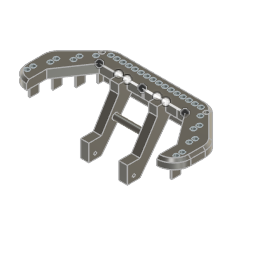
IR Sensor front (Autodesk Fusion 360 design; units mm, degrees)
part number: 2026-02-09-01-24-13-625
Autodesk Fusion 360 part; units mm, degrees
note: some values were not read from the file. Set by a fixed rule: which sketch regions a step uses.
sketch "Sketch1" plane through (0, 0, 0) normal (0, 0, 1) x (1, 0, 0)
  line L0 (0.0284, 49.9803) -> (112.0284, 49.9803)
  line L1 (0.0284, 49.9803) -> (14, 49.9848)
  line L2 (34, 49.9803) -> (35, 49.9803)
  line L3 (0.0284, 49.9803) -> (3.5, 49.981)
  circle A0 centre (3.5, 40) radius 2.5
  circle A1 centre (10.5, 40) radius 2.5
  circle A2 centre (17.5, 40) radius 2.5
  circle A3 centre (24.5, 40) radius 2.5
  circle A4 centre (52.5, 40) radius 2.5
  circle A5 centre (45.5, 40) radius 2.5
  circle A6 centre (38.5, 40) radius 2.5
  circle A7 centre (31.5, 40) radius 2.5
  circle A8 centre (80.5, 40) radius 2.5
  circle A9 centre (66.5, 40) radius 2.5
  circle A10 centre (87.5, 40) radius 2.5
  circle A11 centre (108.5, 40) radius 2.5
  circle A12 centre (101.5, 40) radius 2.5
  circle A13 centre (59.5, 40) radius 2.5
  circle A14 centre (73.5, 40) radius 2.5
  circle A15 centre (94.5, 40) radius 2.5
  line L4 (0.0284, 49.9803) -> (112, 49.9803)
  line L5 (0.0284, 35) -> (18.4391, 35) construction
  line L6 (0.0284, 49.9803) -> (21.4009, 49.9803) construction
  line L7 (0.0284, 49.9803) -> (17.8045, 49.9803) construction
  line L8 (0.0284, 35) -> (16.4184, 35) construction
  line L9 (0.0284, 35) -> (26.651, 35) construction
  line L10 (0.0284, 35) -> (21.4009, 35) construction
  line L11 (0.0284, 49.9803) -> (16.9706, 49.9803) construction
  line L12 (0.0284, 49.9803) -> (-39.8611, 10.0907)
  line L13 (-39.8611, 10.0907) -> (-39.8327, 0)
  line L14 (-39.8327, 0) -> (-39.734, -35)
  line L15 (16.4256, 25) -> (55, 25)
  line L16 (55, 25) -> (56, 25)
  line L17 (-19.9417, -11.3673) -> (-19.9417, -35)
  line L18 (-39.9417, -35) -> (-19.9417, -35)
  line L19 (-19.9417, -11.3673) -> (16.4256, 25)
  line L20 (-19.9417, -11.3673) -> (31.4894, -11.3673) construction
  line L21 (131.9417, -11.3673) -> (95.5744, 25)
  line L22 (111.9716, 49.9803) -> (98, 49.9848)
  line L23 (111.9716, 49.9803) -> (108.5, 49.981)
  line L24 (151.9417, -35) -> (131.9417, -35)
  line L25 (151.8611, 10.0907) -> (151.8327, 0)
  line L26 (78, 49.9803) -> (77, 49.9803)
  line L27 (151.8327, 0) -> (151.8327, -15)
  line L28 (57, 25) -> (56, 25)
  circle A16 centre (59.5, 40) radius 2.5
  circle A17 centre (87.5, 40) radius 2.5
  line L29 (111.9716, 49.9803) -> (95.0294, 49.9803) construction
  circle A18 centre (66.5, 40) radius 2.5
  circle A19 centre (80.5, 40) radius 2.5
  circle A20 centre (108.5, 40) radius 2.5
  line L30 (111.9716, 49.9803) -> (151.8611, 10.0907)
  line L31 (131.9417, -11.3673) -> (131.9417, -35)
  line L32 (111.9716, 49.9803) -> (94.1955, 49.9803) construction
  circle A21 centre (101.5, 40) radius 2.5
  line L33 (111.9716, 35) -> (95.5816, 35) construction
  line L34 (95.5744, 25) -> (57, 25)
  line L35 (131.9417, -11.3673) -> (80.5106, -11.3673) construction
  circle A22 centre (94.5, 40) radius 2.5
  line L36 (111.9716, 35) -> (90.5991, 35) construction
  circle A23 centre (73.5, 40) radius 2.5
  line L37 (111.9716, 49.9803) -> (90.5991, 49.9803) construction
  line L38 (151.8611, 10.0908) -> (151.8327, 0)
  line L39 (151.8327, 0) -> (151.734, -35)
  line L40 (-10.0048, 29.3243) -> (4.6262, 29.3243) construction
  line L41 (-4.8319, 34.4971) -> (-4.8319, 35.4971)
  line L42 (-4.8319, 35.4971) -> (-4.8319, 37.9971)
  circle A24 centre (-4.8319, 37.9971) radius 2.5
  circle A25 centre (-4.8319, 30.9971) radius 2.5
  line L43 (-19.9163, 19.3711) -> (-5.8699, 19.3711) construction
  line L44 (-9.984, 29.3034) -> (4.3283, 29.3034) construction
  circle A26 centre (-24.9502, -2.1627) radius 2.5
  circle A27 centre (-24.9502, 4.8373) radius 2.5
  circle A28 centre (-30.9502, -16.1627) radius 2.5
  circle A29 centre (-30.9502, -23.1627) radius 2.5
  circle A30 centre (-13.9502, 20.8373) radius 2.5
  circle A31 centre (-13.9502, 13.8373) radius 2.5
  circle A32 centre (116.8319, 37.9971) radius 2.5
  circle A33 centre (116.8319, 30.9971) radius 2.5
  line L45 (116.8319, 35.4971) -> (116.8319, 37.9971)
  line L46 (151.8327, 0) -> (151.734, -35)
  line L47 (116.8319, 34.4971) -> (116.8319, 35.4971)
  line L48 (131.9417, -11.3673) -> (131.9417, -35)
  circle A34 centre (142.9502, -23.1627) radius 2.5
  line L49 (151.9417, -35) -> (131.9417, -35)
  circle A35 centre (136.9502, 4.8373) radius 2.5
  circle A36 centre (125.9502, 20.8373) radius 2.5
  circle A37 centre (142.9502, -16.1627) radius 2.5
  line L50 (131.9163, 19.3711) -> (117.8699, 19.3711) construction
  line L51 (151.8611, 10.0907) -> (151.8327, 0)
  circle A38 centre (125.9502, 13.8373) radius 2.5
  circle A39 centre (136.9502, -2.1627) radius 2.5
  point P0 (151.9417, -35)
  point P1 (121.984, 29.3034)
  point P2 (122.0048, 29.3243)
  dimension "d1" = 112
  dimension "d40" = 45
  dimension "d42" = 1
  dimension "d43" = 2.5
  dimension "d44" = 5
  constraint horizontal L0
  constraint coincident L0 L2.start
  constraint coincident L0 L2.end
  constraint horizontal L4
  constraint horizontal L5
  constraint horizontal L6
  constraint horizontal L7
  constraint horizontal L8
  constraint horizontal L9
  constraint horizontal L10
  constraint horizontal L11
  constraint parallel L13 L14
  constraint perpendicular L17 L18
  constraint horizontal L20
  constraint coincident L18 L14.end
  constraint horizontal L40
  constraint vertical L41
  constraint parallel L41 L42
  constraint coincident L42.end A24.centre
  constraint horizontal L43
  constraint horizontal L44
  measures "d1" distance of L0.start L0.end
  measures "d40" angle of L19 L20
  measures "d42" distance of L41.start L41.end
  measures "d43" distance of L41.end L42.end
  measures "d44" diameter of A24
sketch "Sketch2" plane through (0, 0, 0) normal (0, 0, 1) x (1, 0, 0)
extrude "Extrude1" add sketch "Sketch1" against normal blind 10
fillet "Fillet1" radius 20 6 edges at (151.8611, 10.0907, -5) (151.734, -35, -5) (111.9716, 49.9803, -5) (0.0284, 49.9803, -5) (-39.8611, 10.0907, -5) (-39.734, -35, -5)
sketch "Sketch3" plane through (0, 0, 0) normal (0, 0, 1) x (1, 0, 0)
chamfer "Chamfer1" distance 3 angle 45 13 edges at (42.6564, 49.9803, 0) (77.5, 49.9803, 0) (90.8436, 49.9803, 0) (111.341, 48.4579, 0) (131.9047, 30.0472, 0) (150.3261, 9.4575, 0) (151.814, -6.6417, 0) (145.966, -29.1091, 0) (-33.966, -29.1091, 0) (-39.814, -6.6417, 0) (-38.3261, 9.4575, 0) (-19.9047, 30.0472, 0) (0.659, 48.4579, 0)
sketch "Sketch4" plane through (0, 0, 0) normal (0, 0, 1) x (1, 0, 0)
  line L0 (131.9417, -11.3672) -> (105, 25)
  line L1 (105, 25) -> (5, 25)
  line L2 (5, 25) -> (-19.9417, -11.3672)
  line L3 (-19.9417, -11.3672) -> (131.9417, -11.3672)
  constraint horizontal L1
extrude "Extrude2" cut sketch "Sketch4" against normal blind 10
move_face "OffsetFaces1" offset -0.3 32 faces at (-28.4533, -23.2873, -6.6667) (-28.4533, -16.2873, -6.6667) (-22.4533, -2.2873, -6.6667) (-22.4533, 4.7127, -6.6667) (-11.4533, 13.7127, -6.6667) (-11.4533, 20.7127, -6.6667) (-2.3351, 30.8725, -6.6667) (-5.5688, 35.6082, -6.6667) (5.9969, 39.8754, -6.6667) (12.9969, 39.8754, -6.6667) (19.9969, 39.8754, -6.6667) (26.9969, 39.8754, -6.6667) (33.9969, 39.8754, -6.6667) (40.9969, 39.8754, -6.6667) (47.9969, 39.8754, -6.6667) (54.9969, 39.8754, -6.6667) (61.9969, 39.8754, -6.6667) (68.9969, 39.8754, -6.6667) (75.9969, 39.8754, -6.6667) (82.9969, 39.8754, -6.6667) (89.9969, 39.8754, -6.6667) (96.9969, 39.8754, -6.6667) (103.9969, 39.8754, -6.6667) (110.9969, 39.8754, -6.6667) (117.2186, 40.467, -6.6667) (119.3288, 30.8725, -6.6667) (128.4471, 13.7127, -6.6667) (128.4471, 20.7127, -6.6667) (137.6273, 7.2438, -6.6667) (137.6273, 0.2438, -6.6667) (143.6273, -13.7562, -6.6667) (143.6273, -20.7562, -6.6667)
sketch "Sketch5" plane through (0, 0, 0) normal (0, 0, 1) x (1, 0, 0)
sketch "Sketch6" plane through (0, 0, 0) normal (1, 0, 0) x (0, 1, 0)
sketch "Sketch7" plane through (0, 0, 0) normal (0, 0, 1) x (1, 0, 0)
sketch "Sketch8" plane through (0, 0, 0) normal (1, 0, 0) x (0, 1, 0)
sketch "Sketch9" plane through (0, 0, -10) normal (0, 0, -1) x (1, 0, 0)
  circle A0 centre (3.5, -40) radius 2.8
  circle A1 centre (136.9502, -4.8373) radius 2.8
  circle A2 centre (-13.9502, -13.8373) radius 2.8
  circle A3 centre (17.5, -40) radius 2.8
  circle A4 centre (142.9502, 23.1627) radius 2.8
  circle A5 centre (-24.9502, -4.8373) radius 2.8
  circle A6 centre (-13.9502, -20.8373) radius 2.8
  circle A7 centre (73.5, -40) radius 2.8
  circle A8 centre (52.5, -40) radius 2.8
  circle A9 centre (116.8319, -37.9971) radius 2.8
  circle A10 centre (-4.8319, -37.9971) radius 2.8
  circle A11 centre (45.5, -40) radius 2.8
  circle A12 centre (136.9502, 2.1627) radius 2.8
  circle A13 centre (10.5, -40) radius 2.8
  circle A14 centre (-30.9502, 23.1627) radius 2.8
  circle A15 centre (116.8319, -30.9971) radius 2.8
  circle A16 centre (66.5, -40) radius 2.8
  circle A17 centre (24.5, -40) radius 2.8
  circle A18 centre (108.5, -40) radius 2.8
  circle A19 centre (-4.8319, -30.9971) radius 2.8
  circle A20 centre (142.9502, 16.1627) radius 2.8
  circle A21 centre (94.5, -40) radius 2.8
  circle A22 centre (125.9502, -20.8373) radius 2.8
  circle A23 centre (59.5, -40) radius 2.8
  circle A24 centre (31.5, -40) radius 2.8
  circle A25 centre (101.5, -40) radius 2.8
  circle A26 centre (125.9502, -13.8373) radius 2.8
  circle A27 centre (-24.9502, 2.1627) radius 2.8
  circle A28 centre (80.5, -40) radius 2.8
  circle A29 centre (87.5, -40) radius 2.8
  circle A30 centre (38.5, -40) radius 2.8
  circle A31 centre (-30.9502, 16.1627) radius 2.8
  line L0 (131.9417, 11.3673) -> (105, -25)
  line L1 (105, -25) -> (95.5744, -25)
  line L2 (95.5744, -25) -> (57, -25)
  line L3 (57, -25) -> (55, -25)
  line L4 (55, -25) -> (5, -25)
  line L5 (5, -25) -> (-19.9417, 11.3672)
  line L6 (-19.9417, 11.3673) -> (-19.9417, 35)
  arc A32 (-19.9417, 35) -> (-39.7902, 15.057) centre (-19.7903, 15.0006) ccw
  line L7 (-39.7902, 15.057) -> (-39.8377, -1.7735)
  arc A33 (-39.8377, -1.7735) -> (-33.9799, -15.972) centre (-19.8378, -1.8298) ccw
  line L8 (-33.9799, -15.972) -> (-5.8294, -44.1225)
  arc A34 (-5.8294, -44.1225) -> (8.3127, -49.9803) centre (8.3127, -29.9803) ccw
  line L9 (8.3127, -49.9803) -> (77, -49.9803)
  line L10 (77, -49.9803) -> (78, -49.9803)
  line L11 (78, -49.9803) -> (103.6873, -49.9803)
  arc A35 (103.6873, -49.9803) -> (117.8294, -44.1225) centre (103.6873, -29.9803) ccw
  line L12 (117.8294, -44.1225) -> (145.9799, -15.972)
  arc A36 (145.9799, -15.972) -> (151.8377, -1.7735) centre (131.8378, -1.8298) ccw
  line L13 (151.8377, -1.7735) -> (151.7902, 15.057)
  arc A37 (151.7902, 15.057) -> (131.9417, 35) centre (131.7903, 15.0006) ccw
  line L14 (131.9417, 35) -> (131.9417, 11.3673)
  line L15 (111.7359, -34.6155) -> (0, -34.6155)
  line L16 (111.7359, -36.6155) -> (0, -36.6155)
  line L17 (113.7359, -39.4874) -> (113.7359, -28.7703)
  line L18 (111.7359, -39.483) -> (111.7359, -28.6527)
  line L19 (122.7359, -22.5163) -> (122.7359, -11.7992)
  line L20 (120.7359, -22.5119) -> (120.7359, -11.6815)
  line L21 (131.7359, -6.4947) -> (131.7359, 4.3357)
  line L22 (133.7359, -6.4991) -> (133.7359, 4.218)
  line L23 (137.7359, 14.5053) -> (137.7359, 25.3357)
  line L24 (139.7359, 14.5009) -> (139.7359, 25.218)
  line L25 (139.7359, 14.5009) -> (137.7359, 14.5053)
  line L26 (137.7359, 25.3357) -> (139.7359, 25.218)
  line L27 (133.7359, 4.218) -> (131.7359, 4.3357)
  line L28 (131.7359, -6.4947) -> (133.7359, -6.4991)
  line L29 (122.7359, -11.7992) -> (120.7359, -11.6815)
  line L30 (120.7359, -22.5119) -> (122.7359, -22.5163)
  line L31 (113.7359, -28.7703) -> (111.7359, -28.6527)
  line L32 (113.7359, -39.4874) -> (111.7359, -39.483)
  line L33 (56.7001, -39.9767) -> (55.2999, -39.9767)
  line L34 (56, -39.9767) -> (56, -24)
  line L35 (-25.7359, 14.5053) -> (-25.7359, 25.3357)
  line L36 (-27.7359, 14.5009) -> (-27.7359, 25.218)
  line L37 (-27.7359, 14.5009) -> (-25.7359, 14.5053)
  line L38 (-25.7359, 25.3357) -> (-27.7359, 25.218)
  line L39 (-19.7359, -6.4947) -> (-21.7359, -6.4991)
  line L40 (-19.7359, -6.4947) -> (-19.7359, 4.3357)
  line L41 (-21.7359, -6.4991) -> (-21.7359, 4.218)
  line L42 (-21.7359, 4.218) -> (-19.7359, 4.3357)
  line L43 (-8.7359, -22.5119) -> (-8.7359, -11.6815)
  line L44 (-10.7359, -11.7992) -> (-8.7359, -11.6815)
  line L45 (-10.7359, -22.5163) -> (-10.7359, -11.7992)
  line L46 (-8.7359, -22.5119) -> (-10.7359, -22.5163)
  line L47 (0.2641, -39.9767) -> (0.2641, -28.6527)
  line L48 (-1.7359, -28.7703) -> (0.2641, -28.6527)
  line L49 (-1.7359, -39.4874) -> (-1.7359, -28.7703)
  line L50 (-1.7359, -39.4874) -> (0.2641, -39.483)
  dimension "d63" = 2
  dimension "d64" = 2
  dimension "d65" = 2
  constraint horizontal L15
  constraint vertical L17
  constraint coincident L18 L15.start
  constraint vertical L19
  constraint vertical L22
  constraint vertical L24
  constraint parallel L26 L27
  constraint coincident A23 L33.start
  constraint coincident A8 L33.end
  constraint horizontal L33
  constraint midpoint L33 L34.start
  constraint perpendicular L3 L34
  constraint symmetric L17.end L34 L48.start
  constraint symmetric L18.start L34 L50.end
  constraint symmetric L18.end L34 L47.end
  constraint symmetric L17.start L34 L49.start
  constraint symmetric L19.end L34 L44.start
  constraint symmetric L19.start L34 L45.start
  constraint symmetric L20.start L34 L43.start
  constraint symmetric L20.end L34 L43.end
  constraint symmetric L21.start L34 L39.start
  constraint symmetric L21.end L34 L40.end
  constraint symmetric L22.end L34 L41.end
  constraint symmetric L22.start L34 L39.end
  constraint symmetric L24.start L34 L36.start
  constraint symmetric L23.start L34 L35.start
  constraint symmetric L23.end L34 L35.end
  constraint symmetric L24.end L34 L36.end
  constraint coincident L50.end L47
  constraint coincident L18 L16.start
  measures "d63" distance of L19 L20
  measures "d64" distance of L21 L22
  measures "d65" distance of L23 L24
extrude "Extrude3" add sketch "Sketch9" along normal blind 15 contours L15 L16 L18 L34 | L17 L18 L31 L32 | L15 L16 L34 L47 | L47 L48 L49 L50 | L19 L20 L29 L30 | L21 L22 L27 L28 | L23 L24 L25 L26 | L35 L36 L37 L38 | L39 L40 L41 L42 | L43 L44 L45 L46
sketch "Sketch10" plane through (0, 0, 0) normal (0, 0, 1) x (-1, 0, 0)
  line L0 (-105, -25) -> (-131.9417, 11.3673)
  line L1 (-131.9417, 11.3673) -> (-131.9417, 31.9999)
  arc A0 (-131.9417, 31.9999) -> (-148.7902, 15.0485) centre (-131.7903, 15.0006) ccw
  line L2 (-148.7902, 15.0485) -> (-148.8377, -1.7819)
  arc A1 (-148.8377, -1.7819) -> (-143.8586, -13.8507) centre (-131.8378, -1.8298) ccw
  line L3 (-143.8586, -13.8507) -> (-119.6308, -38.0785)
  arc A2 (-116.9133, -40.7959) -> (-119.6308, -38.0785) centre (-116.8319, -37.9971) ccw
  line L4 (-116.9133, -40.7959) -> (-115.7081, -42.0011)
  arc A3 (-115.7081, -42.0011) -> (-103.6873, -46.9803) centre (-103.6873, -29.9803) ccw
  line L5 (-103.6873, -46.9803) -> (-78, -46.9803)
  line L6 (-78, -46.9803) -> (-77, -46.9803)
  line L7 (-77, -46.9803) -> (-8.3127, -46.9803)
  arc A4 (-8.3127, -46.9803) -> (3.7081, -42.0011) centre (-8.3127, -29.9803) ccw
  line L8 (3.7081, -42.0011) -> (4.9133, -40.7959)
  arc A5 (7.6308, -38.0785) -> (4.9133, -40.7959) centre (4.8319, -37.9971) ccw
  line L9 (7.6308, -38.0785) -> (31.8586, -13.8507)
  arc A6 (31.8586, -13.8507) -> (36.8377, -1.7819) centre (19.8378, -1.8298) ccw
  line L10 (36.8377, -1.7819) -> (36.7902, 15.0485)
  arc A7 (36.7902, 15.0485) -> (19.9417, 31.9999) centre (19.7903, 15.0006) ccw
  line L11 (19.9417, 31.9999) -> (19.9417, 11.3673)
  line L12 (19.9417, 11.3672) -> (-5, -25)
  line L13 (-5, -25) -> (-55, -25)
  line L14 (-55, -25) -> (-57, -25)
  line L15 (-57, -25) -> (-95.5744, -25)
  line L16 (-95.5744, -25) -> (-105, -25)
  circle A8 centre (30.9502, 16.1627) radius 2.8
  circle A9 centre (-38.5, -40) radius 2.8
  circle A10 centre (-87.5, -40) radius 2.8
  circle A11 centre (-80.5, -40) radius 2.8
  circle A12 centre (24.9502, 2.1627) radius 2.8
  circle A13 centre (-125.9502, -13.8373) radius 2.8
  circle A14 centre (-101.5, -40) radius 2.8
  circle A15 centre (-31.5, -40) radius 2.8
  circle A16 centre (-59.5, -40) radius 2.8
  circle A17 centre (-125.9502, -20.8373) radius 2.8
  circle A18 centre (-94.5, -40) radius 2.8
  circle A19 centre (-142.9502, 16.1627) radius 2.8
  circle A20 centre (4.8319, -30.9971) radius 2.8
  circle A21 centre (-108.5, -40) radius 2.8
  circle A22 centre (-24.5, -40) radius 2.8
  circle A23 centre (-66.5, -40) radius 2.8
  circle A24 centre (-116.8319, -30.9971) radius 2.8
  circle A25 centre (30.9502, 23.1627) radius 2.8
  circle A26 centre (-10.5, -40) radius 2.8
  circle A27 centre (-136.9502, 2.1627) radius 2.8
  circle A28 centre (-45.5, -40) radius 2.8
  circle A29 centre (-52.5, -40) radius 2.8
  circle A30 centre (-73.5, -40) radius 2.8
  circle A31 centre (13.9502, -20.8373) radius 2.8
  circle A32 centre (24.9502, -4.8373) radius 2.8
  circle A33 centre (-142.9502, 23.1627) radius 2.8
  circle A34 centre (-17.5, -40) radius 2.8
  circle A35 centre (13.9502, -13.8373) radius 2.8
  circle A36 centre (-136.9502, -4.8373) radius 2.8
  circle A37 centre (-3.5, -40) radius 2.8
  line L17 (-5, -25) -> (-105, -25)
  line L18 (-105, -25) -> (-55, -25)
  line L19 (-55, -25) -> (-27.5, -25)
  line L20 (-55, -25) -> (-37.5, -25)
  line L21 (-55, -25) -> (-72.5, -25)
  line L22 (-55, -25) -> (-82.5, -25)
  dimension "d68" = 50
  dimension "d69" = 27.5
  dimension "d70" = 17.5
  dimension "d71" = 17.5
  dimension "d72" = 27.5
  constraint coincident L12.end L13.start
  constraint coincident L0.start L16.end
  constraint parallel L17 L18
  constraint parallel L17 L19
  constraint coincident L13.end L14.start
  constraint parallel L19 L20
  constraint parallel L15 L21
  constraint parallel L17 L22
  measures "d68" distance of L0.start L13.end
  measures "d69" distance of L13.end L19.end
  measures "d70" distance of L13.end L20.end
  measures "d71" distance of L13.end L21.end
  measures "d72" distance of L13.end L22.end
sketch "Sketch11" plane through (0, 25, 0) normal (0, -1, 0) x (1, 0, 0)
  line L0 (95.5744, 0) -> (57, 0)
  line L1 (57, 0) -> (57, -10)
  line L2 (57, -10) -> (95.5744, -10)
  line L3 (95.5744, -10) -> (95.5744, 0)
  line L4 (82.5, 0) -> (72.5, 0)
  line L5 (72.5, 0) -> (72.5, -10)
  line L6 (72.5, -10) -> (82.5, -10)
  line L7 (82.5, -10) -> (82.5, 0)
  line L8 (37.5, 0) -> (27.5, 0)
  line L9 (27.5, 0) -> (27.5, -10)
  line L10 (27.5, -10) -> (37.5, -10)
  line L11 (37.5, -10) -> (37.5, 0)
  point P0 (82.5, 0)
  point P1 (72.5, 0)
  point P2 (37.5, 0)
  point P3 (27.5, 0)
  dimension "d73" = 10
  dimension "d74" = 10
  dimension "d75" = 10
  dimension "d76" = 10
  constraint horizontal L4
  constraint vertical L5
  constraint horizontal L6
  constraint vertical L7
  constraint coincident P0 L4.start
  constraint horizontal L8
  constraint vertical L9
  constraint horizontal L10
  constraint vertical L11
  constraint coincident P2 L8.start
  measures "d73" distance of P0 P1
  measures "d74" distance of P0 L6.end
  measures "d75" distance of P2 P3
  measures "d76" distance of P2 L10.end
ref_plane "WorkPlane1" through (30, -5, -5) normal (0, -1, 0) x (-1, 0, 0)
sketch "Sketch12" plane through (0, -5, 0) normal (0, -1, 0) x (-1, 0, 0)
  line L0 (-37.5, 42) -> (-27.9, 42)
  line L1 (-27.9, 42) -> (-27.9, 62)
  line L2 (-27.9, 62) -> (-37.5, 62)
  line L3 (-37.5, 62) -> (-37.5, 42)
  point P0 (-72.5, 0)
  point P1 (-82.5, 0)
  point P2 (-27.5, 0)
  point P3 (-37.5, 0)
  dimension "d81" = 42
  dimension "d82" = 9.6
  dimension "d83" = 20
  constraint horizontal L0
  constraint vertical L1
  constraint horizontal L2
  constraint vertical L3
  measures "d81" distance of P3 L0.start
  measures "d82" distance of L0.start L0.end
  measures "d83" distance of L0.start L2.end
extrude "Extrude4" add sketch "Sketch11" along normal blind 10 contours L0 L2 L4 L5 L6 L7 | L8 L9 L10 L11
sketch "Sketch13" plane through (0, 0, -10) normal (0, 0, -1) x (1, 0, 0)
  line L0 (-27.7359, 14.5009) -> (-27.7359, 25.218)
  line L1 (-27.7359, 25.218) -> (-25.7359, 25.3357)
  line L2 (-25.7359, 25.3357) -> (-25.7359, 14.5053)
  line L3 (-25.7359, 14.5053) -> (-27.7359, 14.5009)
  line L4 (131.7359, -6.4947) -> (131.7359, 4.3357)
  line L5 (131.7359, 4.3357) -> (133.7359, 4.218)
  line L6 (133.7359, 4.218) -> (133.7359, -6.4991)
  line L7 (133.7359, -6.4991) -> (131.7359, -6.4947)
  line L8 (120.7359, -22.5119) -> (120.7359, -11.6815)
  line L9 (120.7359, -11.6815) -> (122.7359, -11.7992)
  line L10 (122.7359, -11.7992) -> (122.7359, -22.5163)
  line L11 (122.7359, -22.5163) -> (120.7359, -22.5119)
  line L12 (-19.7359, -6.4947) -> (-21.7359, -6.4991)
  line L13 (-21.7359, -6.4991) -> (-21.7359, 4.218)
  line L14 (-21.7359, 4.218) -> (-19.7359, 4.3357)
  line L15 (-19.7359, 4.3357) -> (-19.7359, -6.4947)
  line L16 (139.7359, 14.5009) -> (137.7359, 14.5053)
  line L17 (137.7359, 14.5053) -> (137.7359, 25.3357)
  line L18 (137.7359, 25.3357) -> (139.7359, 25.218)
  line L19 (139.7359, 25.218) -> (139.7359, 14.5009)
  line L20 (-1.7359, -28.7703) -> (0.2641, -28.6527)
  line L21 (0.2641, -28.6527) -> (0.2641, -34.6155)
  line L22 (0.2641, -34.6155) -> (111.7359, -34.6155)
  line L23 (111.7359, -34.6155) -> (111.7359, -28.6527)
  line L24 (111.7359, -28.6527) -> (113.7359, -28.7703)
  line L25 (113.7359, -28.7703) -> (113.7359, -39.4874)
  line L26 (113.7359, -39.4874) -> (111.7359, -39.483)
  line L27 (111.7359, -39.483) -> (111.7359, -36.6155)
  line L28 (111.7359, -36.6155) -> (0.2641, -36.6155)
  line L29 (0.2641, -36.6155) -> (0.2641, -39.483)
  line L30 (0.2641, -39.483) -> (-1.7359, -39.4874)
  line L31 (-1.7359, -39.4874) -> (-1.7359, -28.7703)
  line L32 (-8.7359, -22.5119) -> (-10.7359, -22.5163)
  line L33 (-10.7359, -22.5163) -> (-10.7359, -11.7992)
  line L34 (-10.7359, -11.7992) -> (-8.7359, -11.6815)
  line L35 (-8.7359, -11.6815) -> (-8.7359, -22.5119)
  circle A0 centre (3.5, -40) radius 2.8
  circle A1 centre (136.9502, -4.8373) radius 2.8
  circle A2 centre (-13.9502, -13.8373) radius 2.8
  circle A3 centre (17.5, -40) radius 2.8
  circle A4 centre (142.9502, 23.1627) radius 2.8
  circle A5 centre (-24.9502, -4.8373) radius 2.8
  circle A6 centre (-13.9502, -20.8373) radius 2.8
  circle A7 centre (73.5, -40) radius 2.8
  circle A8 centre (52.5, -40) radius 2.8
  circle A9 centre (116.8319, -37.9971) radius 2.8
  circle A10 centre (-4.8319, -37.9971) radius 2.8
  circle A11 centre (45.5, -40) radius 2.8
  circle A12 centre (136.9502, 2.1627) radius 2.8
  circle A13 centre (10.5, -40) radius 2.8
  circle A14 centre (-30.9502, 23.1627) radius 2.8
  circle A15 centre (116.8319, -30.9971) radius 2.8
  circle A16 centre (66.5, -40) radius 2.8
  circle A17 centre (24.5, -40) radius 2.8
  circle A18 centre (108.5, -40) radius 2.8
  circle A19 centre (-4.8319, -30.9971) radius 2.8
  circle A20 centre (142.9502, 16.1627) radius 2.8
  circle A21 centre (94.5, -40) radius 2.8
  circle A22 centre (125.9502, -20.8373) radius 2.8
  circle A23 centre (59.5, -40) radius 2.8
  circle A24 centre (31.5, -40) radius 2.8
  circle A25 centre (101.5, -40) radius 2.8
  circle A26 centre (125.9502, -13.8373) radius 2.8
  circle A27 centre (-24.9502, 2.1627) radius 2.8
  circle A28 centre (80.5, -40) radius 2.8
  circle A29 centre (87.5, -40) radius 2.8
  circle A30 centre (38.5, -40) radius 2.8
  circle A31 centre (-30.9502, 16.1627) radius 2.8
  line L36 (131.9417, 11.3673) -> (105, -25)
  line L37 (105, -25) -> (95.5744, -25)
  line L38 (95.5744, -25) -> (82.5, -25)
  line L39 (82.5, -25) -> (82.5, -15)
  line L40 (82.5, -15) -> (72.5, -15)
  line L41 (72.5, -15) -> (72.5, -25)
  line L42 (72.5, -25) -> (57, -25)
  line L43 (57, -25) -> (55, -25)
  line L44 (55, -25) -> (37.5, -25)
  line L45 (37.5, -25) -> (37.5, -15)
  line L46 (37.5, -15) -> (27.5, -15)
  line L47 (27.5, -15) -> (27.5, -25)
  line L48 (27.5, -25) -> (5, -25)
  line L49 (5, -25) -> (-19.9417, 11.3672)
  line L50 (-19.9417, 11.3673) -> (-19.9417, 35)
  arc A32 (-19.9417, 35) -> (-39.7902, 15.057) centre (-19.7903, 15.0006) ccw
  line L51 (-39.7902, 15.057) -> (-39.8377, -1.7735)
  arc A33 (-39.8377, -1.7735) -> (-33.9799, -15.972) centre (-19.8378, -1.8298) ccw
  line L52 (-33.9799, -15.972) -> (-5.8294, -44.1225)
  arc A34 (-5.8294, -44.1225) -> (8.3127, -49.9803) centre (8.3127, -29.9803) ccw
  line L53 (8.3127, -49.9803) -> (77, -49.9803)
  line L54 (77, -49.9803) -> (78, -49.9803)
  line L55 (78, -49.9803) -> (103.6873, -49.9803)
  arc A35 (103.6873, -49.9803) -> (117.8294, -44.1225) centre (103.6873, -29.9803) ccw
  line L56 (117.8294, -44.1225) -> (145.9799, -15.972)
  arc A36 (145.9799, -15.972) -> (151.8377, -1.7735) centre (131.8378, -1.8298) ccw
  line L57 (151.8377, -1.7735) -> (151.7902, 15.057)
  arc A37 (151.7902, 15.057) -> (131.9417, 35) centre (131.7903, 15.0006) ccw
  line L58 (131.9417, 35) -> (131.9417, 11.3673)
  line L59 (82.5, -15) -> (72.5, -15)
  line L60 (72.5, -15) -> (72.5, -34.6155)
  line L61 (72.5, -34.6155) -> (82.5, -34.6155)
  line L62 (82.5, -34.6155) -> (82.5, -15)
  line L63 (37.5, -15) -> (27.5, -15)
  line L64 (27.5, -15) -> (27.5, -34.6155)
  line L65 (27.5, -34.6155) -> (37.5, -34.6155)
  line L66 (37.5, -34.6155) -> (37.5, -15)
  dimension "d86" = 10
  dimension "d87" = 10
  constraint horizontal L59
  constraint vertical L60
  constraint horizontal L61
  constraint vertical L62
  constraint coincident L39.end L40.start
  constraint horizontal L63
  constraint vertical L64
  constraint horizontal L65
  constraint vertical L66
  constraint coincident L45.end L46.start
  measures "d86" distance of L39.end L40.end
  measures "d87" distance of L45.end L46.end
sketch "Sketch14" plane through (0, 0, -10) normal (0, 0, -1) x (1, 0, 0)
loft "Loft1" add profiles "Sketch13", "Sketch12" section 1 contours L22 L45 L46 L47 L63 L64 L65 L66 section 2
sketch "Sketch15" plane through (0, 0, -10) normal (0, 0, -1) x (1, 0, 0)
  circle A0 centre (-30.9502, 16.1627) radius 2.8
  circle A1 centre (38.5, -40) radius 2.8
  circle A2 centre (87.5, -40) radius 2.8
  circle A3 centre (80.5, -40) radius 2.8
  circle A4 centre (-24.9502, 2.1627) radius 2.8
  circle A5 centre (125.9502, -13.8373) radius 2.8
  circle A6 centre (101.5, -40) radius 2.8
  circle A7 centre (31.5, -40) radius 2.8
  circle A8 centre (59.5, -40) radius 2.8
  circle A9 centre (125.9502, -20.8373) radius 2.8
  circle A10 centre (94.5, -40) radius 2.8
  circle A11 centre (142.9502, 16.1627) radius 2.8
  circle A12 centre (-4.8319, -30.9971) radius 2.8
  circle A13 centre (108.5, -40) radius 2.8
  circle A14 centre (24.5, -40) radius 2.8
  circle A15 centre (66.5, -40) radius 2.8
  circle A16 centre (116.8319, -30.9971) radius 2.8
  circle A17 centre (-30.9502, 23.1627) radius 2.8
  circle A18 centre (10.5, -40) radius 2.8
  circle A19 centre (136.9502, 2.1627) radius 2.8
  circle A20 centre (45.5, -40) radius 2.8
  circle A21 centre (-4.8319, -37.9971) radius 2.8
  circle A22 centre (116.8319, -37.9971) radius 2.8
  circle A23 centre (52.5, -40) radius 2.8
  circle A24 centre (73.5, -40) radius 2.8
  circle A25 centre (-13.9502, -20.8373) radius 2.8
  circle A26 centre (-24.9502, -4.8373) radius 2.8
  circle A27 centre (142.9502, 23.1627) radius 2.8
  circle A28 centre (17.5, -40) radius 2.8
  circle A29 centre (-13.9502, -13.8373) radius 2.8
  circle A30 centre (136.9502, -4.8373) radius 2.8
  circle A31 centre (3.5, -40) radius 2.8
  line L0 (-8.7359, -22.5119) -> (-10.7359, -22.5163)
  line L1 (-10.7359, -22.5163) -> (-10.7359, -11.7992)
  line L2 (-10.7359, -11.7992) -> (-8.7359, -11.6815)
  line L3 (-8.7359, -11.6815) -> (-8.7359, -22.5119)
  line L4 (37.5, -25) -> (37.5, -34.6155)
  line L5 (37.5, -34.6155) -> (111.7359, -34.6155)
  line L6 (111.7359, -34.6155) -> (111.7359, -28.6527)
  line L7 (111.7359, -28.6527) -> (113.7359, -28.7703)
  line L8 (113.7359, -28.7703) -> (113.7359, -39.4874)
  line L9 (113.7359, -39.4874) -> (111.7359, -39.483)
  line L10 (111.7359, -39.483) -> (111.7359, -36.6155)
  line L11 (111.7359, -36.6155) -> (0.2641, -36.6155)
  line L12 (0.2641, -36.6155) -> (0.2641, -39.483)
  line L13 (0.2641, -39.483) -> (-1.7359, -39.4874)
  line L14 (-1.7359, -39.4874) -> (-1.7359, -28.7703)
  line L15 (-1.7359, -28.7703) -> (0.2641, -28.6527)
  line L16 (0.2641, -28.6527) -> (0.2641, -34.6155)
  line L17 (0.2641, -34.6155) -> (27.5, -34.6155)
  line L18 (27.5, -34.6155) -> (27.5, -25)
  line L19 (27.5, -25) -> (5, -25)
  line L20 (5, -25) -> (-19.9417, 11.3672)
  line L21 (-19.9417, 11.3673) -> (-19.9417, 35)
  arc A32 (-19.9417, 35) -> (-39.7902, 15.057) centre (-19.7903, 15.0006) ccw
  line L22 (-39.7902, 15.057) -> (-39.8377, -1.7735)
  arc A33 (-39.8377, -1.7735) -> (-33.9799, -15.972) centre (-19.8378, -1.8298) ccw
  line L23 (-33.9799, -15.972) -> (-5.8294, -44.1225)
  arc A34 (-5.8294, -44.1225) -> (8.3127, -49.9803) centre (8.3127, -29.9803) ccw
  line L24 (8.3127, -49.9803) -> (77, -49.9803)
  line L25 (77, -49.9803) -> (78, -49.9803)
  line L26 (78, -49.9803) -> (103.6873, -49.9803)
  arc A35 (103.6873, -49.9803) -> (117.8294, -44.1225) centre (103.6873, -29.9803) ccw
  line L27 (117.8294, -44.1225) -> (145.9799, -15.972)
  arc A36 (145.9799, -15.972) -> (151.8377, -1.7735) centre (131.8378, -1.8298) ccw
  line L28 (151.8377, -1.7735) -> (151.7902, 15.057)
  arc A37 (151.7902, 15.057) -> (131.9417, 35) centre (131.7903, 15.0006) ccw
  line L29 (131.9417, 35) -> (131.9417, 11.3673)
  line L30 (131.9417, 11.3673) -> (105, -25)
  line L31 (105, -25) -> (95.5744, -25)
  line L32 (95.5744, -25) -> (82.5, -25)
  line L33 (82.5, -25) -> (82.5, -15)
  line L34 (82.5, -15) -> (72.5, -15)
  line L35 (72.5, -15) -> (72.5, -25)
  line L36 (72.5, -25) -> (57, -25)
  line L37 (57, -25) -> (55, -25)
  line L38 (55, -25) -> (37.5, -25)
  line L39 (139.7359, 14.5009) -> (137.7359, 14.5053)
  line L40 (137.7359, 14.5053) -> (137.7359, 25.3357)
  line L41 (137.7359, 25.3357) -> (139.7359, 25.218)
  line L42 (139.7359, 25.218) -> (139.7359, 14.5009)
  line L43 (-19.7359, -6.4947) -> (-21.7359, -6.4991)
  line L44 (-21.7359, -6.4991) -> (-21.7359, 4.218)
  line L45 (-21.7359, 4.218) -> (-19.7359, 4.3357)
  line L46 (-19.7359, 4.3357) -> (-19.7359, -6.4947)
  line L47 (120.7359, -22.5119) -> (120.7359, -11.6815)
  line L48 (120.7359, -11.6815) -> (122.7359, -11.7992)
  line L49 (122.7359, -11.7992) -> (122.7359, -22.5163)
  line L50 (122.7359, -22.5163) -> (120.7359, -22.5119)
  line L51 (131.7359, -6.4947) -> (131.7359, 4.3357)
  line L52 (131.7359, 4.3357) -> (133.7359, 4.218)
  line L53 (133.7359, 4.218) -> (133.7359, -6.4991)
  line L54 (133.7359, -6.4991) -> (131.7359, -6.4947)
  line L55 (-27.7359, 14.5009) -> (-27.7359, 25.218)
  line L56 (-27.7359, 25.218) -> (-25.7359, 25.3357)
  line L57 (-25.7359, 25.3357) -> (-25.7359, 14.5053)
  line L58 (-25.7359, 14.5053) -> (-27.7359, 14.5009)
  line L59 (82.5, -15) -> (72.5, -15)
  line L60 (72.5, -15) -> (72.5, -34.6155)
  line L61 (72.5, -34.6155) -> (82.5, -34.6155)
  line L62 (82.5, -34.6155) -> (82.5, -15)
  constraint horizontal L59
  constraint vertical L60
  constraint horizontal L61
  constraint vertical L62
  constraint coincident L5 L60.end
  constraint coincident L33.end L34.start
sketch "Sketch16" plane through (0, -5, 0) normal (0, -1, 0) x (1, 0, 0)
  line L0 (37.5, -62) -> (37.5, -42)
  line L1 (37.5, -42) -> (27.9, -42)
  line L2 (27.9, -42) -> (27.9, -62)
  line L3 (27.9, -62) -> (37.5, -62)
  line L4 (82.5, -42) -> (72.5, -42)
  line L5 (72.5, -42) -> (72.5, -62)
  line L6 (72.5, -62) -> (82.5, -62)
  line L7 (82.5, -62) -> (82.5, -42)
  point P0 (82.5, 0)
  dimension "d88" = 42
  dimension "d89" = 10
  dimension "d90" = 20
  constraint horizontal L4
  constraint vertical L5
  constraint horizontal L6
  constraint vertical L7
  measures "d88" distance of P0 L4.start
  measures "d89" distance of L4.start L4.end
  measures "d90" distance of L4.start L6.end
loft "Loft2" add profiles "Sketch15", "Sketch16" section 1 contours L5 L33 L34 L35 L59 L60 L61 L62 section 2 contours L4 L5 L6 L7
sketch "Sketch17" plane through (37.5, 0, 0) normal (1, 0, 0) x (0, 1, 0)
  line L0 (25, -10) -> (25, 0)
  line L1 (25, 0) -> (15, 0)
  line L2 (15, 0) -> (15, -10)
  line L3 (15, -10) -> (-5, -42)
  line L4 (-5, -42) -> (-5, -62)
  line L5 (-5, -62) -> (34.6155, -10)
  line L6 (34.6155, -10) -> (25, -10)
  circle A0 centre (0, -30) radius 5
  dimension "d91" = 10
  measures "d91" diameter of A0
extrude "Extrude6" add 2 faces at (79.1667, -5, -55.3333) (34.3, -5, -52.0615) along direction (0, -1, 0) blind 14.75
sketch "Sketch18" plane through (82.5, 0, 0) normal (1, 0, 0) x (0, 1, 0)
  line L0 (25, -10) -> (25, 0)
  line L1 (25, 0) -> (15, 0)
  line L2 (15, 0) -> (15, -10)
  line L3 (15, -10) -> (-5, -42)
  line L4 (-5, -42) -> (-19.75, -42)
  line L5 (-19.75, -42) -> (-19.75, -62)
  line L6 (-19.75, -62) -> (-5, -62)
  line L7 (-5, -62) -> (34.6155, -10)
  line L8 (34.6155, -10) -> (25, -10)
  line L9 (-19.75, -42) -> (-12.25, -42)
  line L10 (-12.25, -42) -> (-12.25, -56)
  line L11 (-12.25, -56) -> (-19.75, -56)
  line L12 (-19.75, -56) -> (-19.75, -42)
  circle A0 centre (-32.25, -56) radius 1.6
  dimension "d96" = 7.5
  dimension "d97" = 14
  dimension "d98" = 3.2
  constraint horizontal L9
  constraint vertical L10
  constraint horizontal L11
  constraint vertical L12
  constraint coincident L4.end L5.start
  constraint coincident L10.end L11.start
  measures "d96" distance of L4.end L9.end
  measures "d97" distance of L4.end L11.end
  measures "d98" diameter of A0
sketch "Sketch19" plane through (82.5, 0, 0) normal (1, 0, 0) x (0, 1, 0)
  line L0 (25, -10) -> (25, 0)
  line L1 (25, 0) -> (15, 0)
  line L2 (15, 0) -> (15, -10)
  line L3 (15, -10) -> (-5, -42)
  line L4 (-5, -42) -> (-19.75, -42)
  line L5 (-19.75, -42) -> (-19.75, -62)
  line L6 (-19.75, -62) -> (-5, -62)
  line L7 (-5, -62) -> (34.6155, -10)
  line L8 (34.6155, -10) -> (25, -10)
  line L9 (-19.75, -42) -> (-12.25, -42)
  line L10 (-12.25, -42) -> (-12.25, -56)
  line L11 (-12.25, -56) -> (-19.75, -56)
  line L12 (-19.75, -56) -> (-19.75, -42)
  circle A0 centre (-12.25, -56) radius 1.6
  dimension "d101" = 7.5
  dimension "d102" = 14
  dimension "d103" = 3.2
  constraint horizontal L9
  constraint vertical L10
  constraint horizontal L11
  constraint vertical L12
  constraint coincident L4.end L5.start
  constraint coincident L10.end L11.start
  measures "d101" distance of L4.end L9.end
  measures "d102" distance of L4.end L11.end
  measures "d103" diameter of A0
extrude "Extrude8" cut sketch "Sketch19" against normal blind 100 contours L10 L11 A0 | L10 L11 A0
sketch "Sketch20" plane through (37.5, 0, 0) normal (1, 0, 0) x (0, 1, 0)
  circle A0 centre (-12.25, -56) radius 1.6
  line L0 (25, -10) -> (25, 0)
  line L1 (25, 0) -> (15, 0)
  line L2 (15, 0) -> (15, -10)
  line L3 (15, -10) -> (-5, -42)
  line L4 (-5, -42) -> (-19.75, -42)
  line L5 (-19.75, -42) -> (-19.75, -62)
  line L6 (-19.75, -62) -> (-5, -62)
  line L7 (-5, -62) -> (34.6155, -10)
  line L8 (34.6155, -10) -> (25, -10)
  circle A1 centre (11.2487, -30.3571) radius 3.6484
extrude "Extrude9" add sketch "Sketch20" along normal blind 35 contours A1
